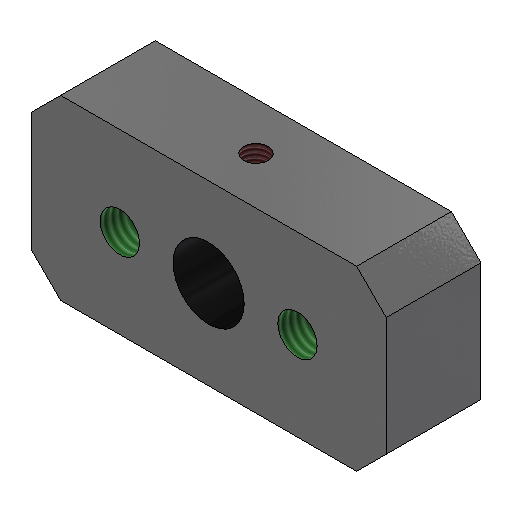
# Autodesk Inventor part: TL20240701-10120CV-023
Saved by Autodesk Inventor 2022.5 (Build 265521000, 521)
## iProperties
Category: FOLLOWER UNIT ASSY
Company: 현대 트랜시스(대유)
Created: 2023-04-11
Part Number: TL20240701-10120CV-023
Checked By: 김형민
Engr Approved By: 김시현
User Status: 2 x18
Material: SS400
Description: 0
Document SubType Name: Modeling
Mfg Approved By: 호상태
Designer: 박성규
Stock Number: 023
Density: 7.85 g/cm^3
Appearance: Plating Zinc White
Project: SW PJT
DETAIL: Coveryor Assembly
M/C TITLE: CJ 제일제당 협동로봇 포장시스탬 PILOT 장비
PARTS NAME: Bracket
SPECIFICATION: TA20221101-CV200000-015
DocNumber: 221118_Standard_v1
Folder: .\
VDS_Category: 엔지니어링
Detail Description: Processed products
Title: BLOCK
Subject: SW차종 시트조립라인
Author: 박성규
Revision Number: A
Autodesk Inventor part; units mm, degrees
ref_plane "YZ Plane" through (0, 0, 0) normal (1, 0, 0) x (0, 1, 0)
ref_plane "XZ Plane" through (0, 0, 0) normal (0, 1, 0) x (-1, 0, 0)
ref_plane "XY Plane" through (0, 0, 0) normal (0, 0, 1) x (1, 0, 0)
sketch "스케치9" plane through (0, 0, 0) normal (0, 0, 1) x (1, 0, 0)
  line L0 (-30, 15) -> (30, 15)
  line L1 (30, 15) -> (30, -15)
  line L2 (30, -15) -> (-30, -15)
  line L3 (-30, -15) -> (-30, 15)
  line L4 (-30, 15) -> (30, -15) construction
  line L5 (30, 15) -> (-30, -15) construction
  point P0 (0, 0)
  dimension "d40" = 30
  dimension "d41" = 60
  constraints: 12 end point, 2 midpoint, 2 parallel, 1 horizontal, 1 perpendicular
  measures "d40" distance of L0.end L1.end
  measures "d41" distance of L0.start L0.end
extrude "돌출4" add sketch "스케치9" along normal blind 16
sketch "스케치10" plane through (0, 0, 16) normal (0, 0, 1) x (1, 0, 0)
  point P0 (0, 0)
  point P1 (0, 0)
  constraints: 1 coincident
hole "구멍3" at (0, 0, 16) direction (0, 0, -1) diameter 12 end through all
sketch "스케치11" plane through (0, 0, 16) normal (0, 0, 1) x (1, 0, 0)
  circle A0 centre (0, 0) radius 6 construction
  point P0 (-15, 0)
  point P1 (15, 0)
  dimension "d51" = 30
  dimension "d52" = 15
  constraints: 2 horizontal alignment
  measures "d51" distance of point (15, 0) point (-15, 0)
  measures "d52" distance of A0.centre point (-15, 0)
hole "구멍4" at (-15, 0, 16) at (15, 0, 16) direction (0, 0, -1) diameter 6.647 end through all thread size "M8x1.25" class "6H" standard "ISO Metric profile"
chamfer "모따기1" distance 5 angle 45 4 edges at (-30, 15, 8) (-30, -15, 8) (30, 15, 8) (30, -15, 8)
sketch "스케치13" plane through (-25, 15, 0) normal (0, 1, 0) x (1, 0, 0)
  line L0 (55, -16) -> (55, 0) projected
  line L1 (50, 0) -> (0, 0) projected
  point P0 (25, 0)
  point P1 (25, -8)
  point P2 (55, -8)
  dimension "d73" = 30
  dimension "d74" = 8
  constraints: 1 midpoint
  measures "d73" distance of point (55, -8) point (25, -8)
  measures "d74" distance from line of point (25, -8) L1
hole "구멍6" at (0, 15, 8) direction (0, -1, 0) diameter 4.134 depth 15 tip angle 118 thread size "M5x0.8" class "6H" standard "ANSI Metric M Profile"
